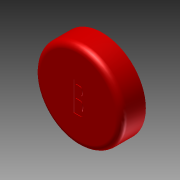
# Autodesk Inventor part: B Button
Saved by Autodesk Inventor 2012 SP1 (Build 160190100, 190)
## iProperties
Created: 2011-11-23
Part Number: B Button
Material: Default
Document SubType Name: Modeling
Designer: 133098
Density: 1 g/cm^3
Author: 133098
Autodesk Inventor part; units mm, degrees
ref_plane "YZ Plane" through (0, 0, 0) normal (1, 0, 0) x (0, 1, 0)
ref_plane "XZ Plane" through (0, 0, 0) normal (0, 1, 0) x (-1, 0, 0)
ref_plane "XY Plane" through (0, 0, 0) normal (0, 0, 1) x (1, 0, 0)
sketch "Sketch1" plane through (0, 0, 0) normal (0, 0, 1) x (1, 0, 0)
  circle A0 centre (0, 0) radius 4.572
  dimension "d0" = 9.144
  constraints: 1 centre point, 1 coincident
  measures "d0" diameter of A0
extrude "Extrusion1" add sketch "Sketch1" along normal blind 2.54
fillet "Fillet1" radius 0.635 1 edges at (-4.572, 0, 2.54)
sketch "Sketch2" plane through (0, 0, 2.54) normal (0, 0, 1) x (1, 0, 0)
  line L0 (-0.5978, 1.4024) -> (2.1711, 1.4024) construction
  line L1 (2.1711, 1.4024) -> (2.1711, -1.6456) construction
  line L2 (2.1711, -1.6456) -> (-0.5978, -1.6456) construction
  line L3 (-0.5978, -1.6456) -> (-0.5978, 1.4024) construction
  line L4 (-0.4421, -1.6456) -> (-0.4421, 1.4024)
  line L5 (-0.4421, 1.4024) -> (0.1271, 1.4024)
  spline S0 degree 2 poles (0.1271, 1.4024) (0.3013, 1.4024) (0.5127, 1.2166) (0.6312, 0.8332) (0.6312, 0.6218) knots 0 0 0 1 2 3 3 3
  spline S1 degree 2 poles (0.6312, 0.6218) (0.6312, 0.4267) (0.5267, 0.0829) (0.4198, -0.024) knots 0 0 0 1 2 2 2
  spline S2 degree 2 poles (0.4198, -0.024) (0.5569, -0.1053) (0.7055, -0.4956) (0.7055, -0.7628) knots 0 0 0 1 2 2 2
  spline S3 degree 2 poles (0.7055, -0.7628) (0.7055, -0.9765) (0.6149, -1.3436) (0.4825, -1.5434) (0.2827, -1.6456) (0.1364, -1.6456) knots 0 0 0 1 2 3 4 4 4
  line L6 (0.1364, -1.6456) -> (-0.4421, -1.6456)
  line L7 (-0.24, -1.2855) -> (0.1387, -1.2855)
  spline S4 degree 2 poles (0.1387, -1.2855) (0.2363, -1.2855) (0.2758, -1.2716) knots 0 0 0 1 1 1
  spline S5 degree 2 poles (0.2758, -1.2716) (0.3455, -1.246) (0.4384, -1.1298) (0.4988, -0.9068) (0.4988, -0.7605) knots 0 0 0 1 2 3 3 3
  spline S6 degree 2 poles (0.4988, -0.7605) (0.4988, -0.5909) (0.4105, -0.34) (0.2549, -0.2377) (0.1108, -0.2377) knots 0 0 0 1 2 3 3 3
  line L8 (0.1108, -0.2377) -> (-0.24, -0.2377)
  line L9 (-0.24, -0.2377) -> (-0.24, -1.2855)
  line L10 (-0.24, 0.1224) -> (0.0876, 0.1224)
  spline S7 degree 2 poles (0.0876, 0.1224) (0.2223, 0.1224) (0.2804, 0.1572) knots 0 0 0 1 1 1
  spline S8 degree 2 poles (0.2804, 0.1572) (0.3571, 0.2037) (0.4337, 0.4151) (0.4337, 0.5754) knots 0 0 0 1 2 2 2
  spline S9 degree 2 poles (0.4337, 0.5754) (0.4337, 0.7264) (0.3617, 0.9564) (0.227, 1.0423) (0.0644, 1.0423) knots 0 0 0 1 2 3 3 3
  line L11 (0.0644, 1.0423) -> (-0.24, 1.0423)
  line L12 (-0.24, 1.0423) -> (-0.24, 0.1224)
  constraints: 2 other
extrude "Extrusion2" cut sketch "Sketch2" against normal blind 0.0635
body "Solid1"
